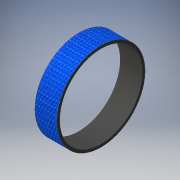
# Autodesk Inventor part: 4InchRoughTopTread(1inWidth)-1111-2017
Saved by Autodesk Inventor 2016 (Build 200138000, 138)
## iProperties
Created: 2017-02-05
Part Number: 4InchRoughTopTread(1inWidth)-1111-2017
Material: Rubber
Document SubType Name: Modeling
Designer: smiku
Density: 0.93 g/cm^3
Appearance: Rubber - Black
Author: smiku
Autodesk Inventor part; units mm, degrees
ref_plane "YZ Plane" through (0, 0, 0) normal (1, 0, 0) x (0, 1, 0)
ref_plane "XZ Plane" through (0, 0, 0) normal (0, 1, 0) x (-1, 0, 0)
ref_plane "XY Plane" through (0, 0, 0) normal (0, 0, 1) x (1, 0, 0)
sketch "Sketch1" plane through (0, 0, 0) normal (1, 0, 0) x (0, 1, 0)
  circle A0 centre (0, 0) radius 47.625
  circle A1 centre (0, 0) radius 50.8
  dimension "d0" = 95.25
  dimension "d1" = 3.175
  dimension "d4" = 101.6
  constraints: 2 centre point, 1 coincident
  measures "d0" diameter of A0
  measures "d1" radial gap between concentric circles of A0 A1
  measures "d4" diameter of A1
extrude "Extrusion1" add sketch "Sketch1" along normal blind 25.4
body "Solid1"
